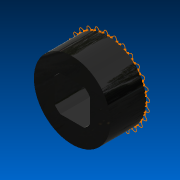
# Autodesk Inventor part: Versa Encoder Adapter
Saved by Autodesk Inventor 2022 (Build 260153000, 153)
## iProperties
Created: 2022-04-19
Part Number: Versa Encoder Adapter
Material: PET Plastic
Document SubType Name: Modeling
Designer: score_nygvs6w
Density: 1.541 g/cm^3
Appearance: Smooth - Black
Author: score_nygvs6w
Autodesk Inventor part; units mm, degrees
ref_plane "YZ Plane" through (0, 0, 0) normal (1, 0, 0) x (0, 1, 0)
ref_plane "XZ Plane" through (0, 0, 0) normal (0, 1, 0) x (-1, 0, 0)
ref_plane "XY Plane" through (0, 0, 0) normal (0, 0, 1) x (1, 0, 0)
sketch "Sketch1" plane through (0, 0, 0) normal (0, 0, 1) x (1, 0, 0)
  point P0 (0, 0)
sketch "Sketch2" plane through (0, 0, 0) normal (0, 0, 1) x (1, 0, 0)
  line L0 (-2.1061, 3.175) -> (2.1061, 3.175)
  line L1 (3.175, 2.1061) -> (3.175, -2.1061)
  line L2 (2.1061, -3.175) -> (-2.1061, -3.175)
  line L3 (-3.175, -2.1061) -> (-3.175, 2.1061)
  arc A0 (-2.1061, 3.175) -> (-3.175, 2.1061) centre (0, 0) ccw
  arc A1 (3.175, 2.1061) -> (2.1061, 3.175) centre (0, 0) ccw
  arc A2 (-3.175, -2.1061) -> (-2.1061, -3.175) centre (0, 0) ccw
  arc A3 (2.1061, -3.175) -> (3.175, -2.1061) centre (0, 0) ccw
  circle A4 centre (0, 0) radius 6.797
  dimension "d0" = 6.35
  dimension "d2" = 3.81
  dimension "d3" = 13.594
  constraints: 8 end point, 8 point on circle, 5 centre point, 4 perpendicular, 3 concentric, 2 coincident, 2 parallel, 1 horizontal
  measures "d0" distance between parallel lines of L1 L3
  measures "d2" radius of A2
  measures "d3" diameter of A4
extrude "Extrusion1" add sketch "Sketch2" along normal blind 6.35
sketch "Sketch3" plane through (0, 0, 0) normal (0, 0, -1) x (-1, 0, 0)
  arc A0 (5.3745, -4.161) -> (5.6838, -3.7274) centre (0, 0) ccw projected
  spline S0 degree 3 poles (5.6838, -3.7274) (5.7254, -3.7321) (5.7892, -3.7379) (5.876, -3.7432) (5.9447, -3.7461) (6.0157, -3.7477) (6.0892, -3.7479) (6.165, -3.7467) (6.2568, -3.7428) (6.3283, -3.7405) (6.3775, -3.7345) (6.39, -3.7308) (6.4012, -3.726) (6.4118, -3.7198) (6.4215, -3.7124) (6.4326, -3.7017) (6.4476, -3.6797) (6.4651, -3.6465) (6.4877, -3.6071) (6.5092, -3.5672) (6.5282, -3.5348) (6.539, -3.5104) (6.5422, -3.4953) (6.5434, -3.4831) (6.543, -3.4709) (6.5411, -3.4589) (6.5377, -3.4463) (6.5169, -3.4013) (6.4811, -3.3394) (6.436, -3.2593) (6.397, -3.1943) (6.3581, -3.132) (6.3192, -3.0725) (6.2805, -3.0157) (6.2301, -2.9448) (6.1916, -2.8937) (6.1656, -2.8608) knots 0.000063 0.000063 0.000063 0.000063 0.072335 0.110531 0.150078 0.190978 0.23323 0.276835 0.321791 0.391759 0.40017 0.407178 0.414186 0.421194 0.428201 0.435209 0.447802 0.473901 0.5 0.526099 0.552198 0.564791 0.571799 0.578806 0.585814 0.592822 0.59983 0.608241 0.678209 0.723165 0.76677 0.809022 0.849922 0.889469 0.927665 0.999937 0.999937 0.999937 0.999937 projected
  arc A1 (6.1656, -2.8608) -> (6.3707, -2.3692) centre (0, 0) ccw projected
  spline S1 degree 3 poles (6.3707, -2.3692) (6.4123, -2.3645) (6.4758, -2.3559) (6.5616, -2.3419) (6.6292, -2.3294) (6.6989, -2.3151) (6.7705, -2.299) (6.8442, -2.281) (6.9328, -2.2567) (7.0019, -2.2386) (7.0486, -2.2217) (7.0599, -2.2153) (7.0698, -2.2081) (7.0787, -2.1998) (7.0866, -2.1904) (7.0951, -2.1775) (7.1048, -2.1527) (7.1145, -2.1164) (7.1277, -2.073) (7.1398, -2.0293) (7.1511, -1.9935) (7.1562, -1.9673) (7.156, -1.9519) (7.1544, -1.9398) (7.1513, -1.9279) (7.1468, -1.9166) (7.1407, -1.9051) (7.1103, -1.8659) (7.0617, -1.8134) (6.9999, -1.7455) (6.9474, -1.6908) (6.8956, -1.6387) (6.8445, -1.5893) (6.7941, -1.5425) (6.7292, -1.4846) (6.6802, -1.4434) (6.6476, -1.4171) knots 0.000063 0.000063 0.000063 0.000063 0.072335 0.110531 0.150078 0.190978 0.23323 0.276835 0.321791 0.391759 0.40017 0.407178 0.414186 0.421194 0.428201 0.435209 0.447802 0.473901 0.5 0.526099 0.552198 0.564791 0.571799 0.578806 0.585814 0.592822 0.59983 0.608241 0.678209 0.723165 0.76677 0.809022 0.849922 0.889469 0.927665 0.999937 0.999937 0.999937 0.999937 projected
  arc A2 (6.6476, -1.4171) -> (6.7382, -0.8922) centre (0, 0) ccw projected
  spline S2 degree 3 poles (6.7382, -0.8922) (6.7777, -0.8783) (6.8377, -0.8559) (6.9182, -0.8231) (6.9813, -0.7959) (7.0461, -0.7665) (7.1123, -0.7347) (7.1801, -0.7008) (7.2611, -0.6575) (7.3245, -0.6244) (7.3662, -0.5976) (7.3759, -0.5888) (7.3839, -0.5796) (7.3908, -0.5695) (7.3963, -0.5586) (7.4017, -0.5441) (7.4056, -0.5178) (7.407, -0.4803) (7.4103, -0.435) (7.4123, -0.3897) (7.4154, -0.3523) (7.4145, -0.3256) (7.4109, -0.3106) (7.4066, -0.2991) (7.401, -0.2883) (7.3941, -0.2782) (7.3856, -0.2684) (7.3472, -0.2369) (7.2882, -0.1966) (7.2128, -0.1441) (7.1495, -0.1024) (7.0874, -0.0632) (7.0265, -0.0264) (6.967, 0.008) (6.8909, 0.05) (6.8339, 0.0793) (6.7963, 0.0977) knots 0.000063 0.000063 0.000063 0.000063 0.072335 0.110531 0.150078 0.190978 0.23323 0.276835 0.321791 0.391759 0.40017 0.407178 0.414186 0.421194 0.428201 0.435209 0.447802 0.473901 0.5 0.526099 0.552198 0.564791 0.571799 0.578806 0.585814 0.592822 0.59983 0.608241 0.678209 0.723165 0.76677 0.809022 0.849922 0.889469 0.927665 0.999937 0.999937 0.999937 0.999937 projected
  arc A3 (6.7963, 0.0977) -> (6.7678, 0.6296) centre (0, 0) ccw projected
  spline S3 degree 3 poles (6.7678, 0.6296) (6.8032, 0.6519) (6.8567, 0.6871) (6.9279, 0.737) (6.9834, 0.7776) (7.04, 0.8207) (7.0975, 0.8663) (7.1561, 0.9145) (7.2254, 0.9748) (7.2798, 1.0212) (7.3145, 1.0566) (7.322, 1.0673) (7.3278, 1.078) (7.3322, 1.0894) (7.3352, 1.1012) (7.3372, 1.1166) (7.3352, 1.1431) (7.3282, 1.18) (7.3213, 1.2249) (7.3132, 1.2695) (7.3078, 1.3067) (7.3011, 1.3324) (7.2942, 1.3463) (7.2875, 1.3565) (7.2796, 1.3658) (7.2706, 1.3741) (7.2601, 1.3818) (7.2157, 1.404) (7.1492, 1.4301) (7.064, 1.4645) (6.993, 1.491) (6.9237, 1.5155) (6.8562, 1.5378) (6.7905, 1.5581) (6.707, 1.5821) (6.6449, 1.598) (6.6042, 1.6076) knots 0.000063 0.000063 0.000063 0.000063 0.072335 0.110531 0.150078 0.190978 0.23323 0.276835 0.321791 0.391759 0.40017 0.407178 0.414186 0.421194 0.428201 0.435209 0.447802 0.473901 0.5 0.526099 0.552198 0.564791 0.571799 0.578806 0.585814 0.592822 0.59983 0.608241 0.678209 0.723165 0.76677 0.809022 0.849922 0.889469 0.927665 0.999937 0.999937 0.999937 0.999937 projected
  arc A4 (6.6042, 1.6076) -> (6.458, 2.1198) centre (0, 0) ccw projected
  spline S4 degree 3 poles (6.458, 2.1198) (6.4876, 2.1494) (6.5319, 2.1956) (6.5902, 2.2601) (6.6353, 2.312) (6.6809, 2.3666) (6.7268, 2.4239) (6.7731, 2.4839) (6.8273, 2.5581) (6.87, 2.6155) (6.896, 2.6577) (6.9009, 2.6698) (6.9042, 2.6816) (6.9059, 2.6936) (6.9062, 2.7058) (6.9048, 2.7213) (6.8969, 2.7467) (6.8819, 2.7811) (6.8652, 2.8233) (6.8474, 2.865) (6.8338, 2.9) (6.8216, 2.9237) (6.8117, 2.9356) (6.8029, 2.9441) (6.7932, 2.9514) (6.7826, 2.9575) (6.7706, 2.9627) (6.7224, 2.9744) (6.6517, 2.9851) (6.561, 2.9997) (6.4859, 3.0097) (6.4129, 3.0182) (6.3421, 3.0249) (6.2736, 3.0301) (6.1867, 3.0349) (6.1227, 3.0366) (6.0809, 3.0368) knots 0.000063 0.000063 0.000063 0.000063 0.072335 0.110531 0.150078 0.190978 0.23323 0.276835 0.321791 0.391759 0.40017 0.407178 0.414186 0.421194 0.428201 0.435209 0.447802 0.473901 0.5 0.526099 0.552198 0.564791 0.571799 0.578806 0.585814 0.592822 0.59983 0.608241 0.678209 0.723165 0.76677 0.809022 0.849922 0.889469 0.927665 0.999937 0.999937 0.999937 0.999937 projected
  arc A5 (6.0809, 3.0368) -> (5.8244, 3.5036) centre (0, 0) ccw projected
  spline S5 degree 3 poles (5.8244, 3.5036) (5.8466, 3.5391) (5.8795, 3.5941) (5.922, 3.6699) (5.9544, 3.7306) (5.9867, 3.7939) (6.0188, 3.86) (6.0506, 3.9288) (6.0869, 4.0132) (6.1158, 4.0786) (6.1317, 4.1256) (6.1338, 4.1385) (6.1344, 4.1506) (6.1334, 4.1628) (6.131, 4.1748) (6.1261, 4.1895) (6.1128, 4.2125) (6.0905, 4.2427) (6.0648, 4.2802) (6.0382, 4.3169) (6.0172, 4.348) (5.9999, 4.3683) (5.9877, 4.3778) (5.9772, 4.3841) (5.9661, 4.3891) (5.9544, 4.3926) (5.9416, 4.395) (5.892, 4.3957) (5.8207, 4.3904) (5.729, 4.3845) (5.6535, 4.3775) (5.5805, 4.3695) (5.51, 4.3603) (5.442, 4.3501) (5.3563, 4.3355) (5.2935, 4.3229) (5.2526, 4.3138) knots 0.000063 0.000063 0.000063 0.000063 0.072335 0.110531 0.150078 0.190978 0.23323 0.276835 0.321791 0.391759 0.40017 0.407178 0.414186 0.421194 0.428201 0.435209 0.447802 0.473901 0.5 0.526099 0.552198 0.564791 0.571799 0.578806 0.585814 0.592822 0.59983 0.608241 0.678209 0.723165 0.76677 0.809022 0.849922 0.889469 0.927665 0.999937 0.999937 0.999937 0.999937 projected
  arc A6 (5.2526, 4.3138) -> (4.8987, 4.7119) centre (0, 0) ccw projected
  spline S6 degree 3 poles (4.8987, 4.7119) (4.9125, 4.7514) (4.9324, 4.8123) (4.9569, 4.8957) (4.975, 4.962) (4.9924, 5.031) (5.0089, 5.1025) (5.0246, 5.1767) (5.0413, 5.2671) (5.0549, 5.3372) (5.06, 5.3866) (5.0591, 5.3996) (5.0569, 5.4116) (5.0533, 5.4233) (5.0483, 5.4344) (5.0403, 5.4476) (5.0221, 5.4672) (4.9937, 5.4916) (4.9603, 5.5224) (4.9262, 5.5523) (4.8988, 5.5779) (4.8775, 5.5939) (4.8634, 5.6004) (4.8518, 5.6042) (4.8399, 5.6066) (4.8277, 5.6075) (4.8146, 5.6069) (4.7661, 5.5966) (4.6978, 5.5756) (4.6098, 5.5494) (4.5377, 5.5258) (4.4683, 5.5017) (4.4016, 5.4771) (4.3376, 5.452) (4.2573, 5.4187) (4.1989, 5.3924) (4.161, 5.3745) knots 0.000063 0.000063 0.000063 0.000063 0.072335 0.110531 0.150078 0.190978 0.23323 0.276835 0.321791 0.391759 0.40017 0.407178 0.414186 0.421194 0.428201 0.435209 0.447802 0.473901 0.5 0.526099 0.552198 0.564791 0.571799 0.578806 0.585814 0.592822 0.59983 0.608241 0.678209 0.723165 0.76677 0.809022 0.849922 0.889469 0.927665 0.999937 0.999937 0.999937 0.999937 projected
  arc A7 (4.161, 5.3745) -> (3.7274, 5.6838) centre (0, 0) ccw projected
  spline S7 degree 3 poles (3.7274, 5.6838) (3.7321, 5.7254) (3.7379, 5.7892) (3.7432, 5.876) (3.7461, 5.9447) (3.7477, 6.0157) (3.7479, 6.0892) (3.7467, 6.165) (3.7428, 6.2568) (3.7405, 6.3283) (3.7345, 6.3775) (3.7308, 6.39) (3.726, 6.4012) (3.7198, 6.4118) (3.7124, 6.4215) (3.7017, 6.4326) (3.6797, 6.4476) (3.6465, 6.4651) (3.6071, 6.4877) (3.5672, 6.5092) (3.5348, 6.5282) (3.5104, 6.539) (3.4953, 6.5422) (3.4831, 6.5434) (3.4709, 6.543) (3.4589, 6.5411) (3.4463, 6.5377) (3.4013, 6.5169) (3.3394, 6.4811) (3.2593, 6.436) (3.1943, 6.397) (3.132, 6.3581) (3.0725, 6.3192) (3.0157, 6.2805) (2.9448, 6.2301) (2.8937, 6.1916) (2.8608, 6.1656) knots 0.000063 0.000063 0.000063 0.000063 0.072335 0.110531 0.150078 0.190978 0.23323 0.276835 0.321791 0.391759 0.40017 0.407178 0.414186 0.421194 0.428201 0.435209 0.447802 0.473901 0.5 0.526099 0.552198 0.564791 0.571799 0.578806 0.585814 0.592822 0.59983 0.608241 0.678209 0.723165 0.76677 0.809022 0.849922 0.889469 0.927665 0.999937 0.999937 0.999937 0.999937 projected
  arc A8 (2.8608, 6.1656) -> (2.3692, 6.3707) centre (0, 0) ccw projected
  spline S8 degree 3 poles (2.3692, 6.3707) (2.3645, 6.4123) (2.3559, 6.4758) (2.3419, 6.5616) (2.3294, 6.6292) (2.3151, 6.6989) (2.299, 6.7705) (2.281, 6.8442) (2.2567, 6.9328) (2.2386, 7.0019) (2.2217, 7.0486) (2.2153, 7.0599) (2.2081, 7.0698) (2.1998, 7.0787) (2.1904, 7.0866) (2.1775, 7.0951) (2.1527, 7.1048) (2.1164, 7.1145) (2.073, 7.1277) (2.0293, 7.1398) (1.9935, 7.1511) (1.9673, 7.1562) (1.9519, 7.156) (1.9398, 7.1544) (1.9279, 7.1513) (1.9166, 7.1468) (1.9051, 7.1407) (1.8659, 7.1103) (1.8134, 7.0617) (1.7455, 6.9999) (1.6908, 6.9474) (1.6387, 6.8956) (1.5893, 6.8445) (1.5425, 6.7941) (1.4846, 6.7292) (1.4434, 6.6802) (1.4171, 6.6476) knots 0.000063 0.000063 0.000063 0.000063 0.072335 0.110531 0.150078 0.190978 0.23323 0.276835 0.321791 0.391759 0.40017 0.407178 0.414186 0.421194 0.428201 0.435209 0.447802 0.473901 0.5 0.526099 0.552198 0.564791 0.571799 0.578806 0.585814 0.592822 0.59983 0.608241 0.678209 0.723165 0.76677 0.809022 0.849922 0.889469 0.927665 0.999937 0.999937 0.999937 0.999937 projected
  arc A9 (1.4171, 6.6476) -> (0.8922, 6.7382) centre (0, 0) ccw projected
  spline S9 degree 3 poles (0.8922, 6.7382) (0.8783, 6.7777) (0.8559, 6.8377) (0.8231, 6.9182) (0.7959, 6.9813) (0.7665, 7.0461) (0.7347, 7.1123) (0.7008, 7.1801) (0.6575, 7.2611) (0.6244, 7.3245) (0.5976, 7.3662) (0.5888, 7.3759) (0.5796, 7.3839) (0.5695, 7.3908) (0.5586, 7.3963) (0.5441, 7.4017) (0.5178, 7.4056) (0.4803, 7.407) (0.435, 7.4103) (0.3897, 7.4123) (0.3523, 7.4154) (0.3256, 7.4145) (0.3106, 7.4109) (0.2991, 7.4066) (0.2883, 7.401) (0.2782, 7.3941) (0.2684, 7.3856) (0.2369, 7.3472) (0.1966, 7.2882) (0.1441, 7.2128) (0.1024, 7.1495) (0.0632, 7.0874) (0.0264, 7.0265) (-0.008, 6.967) (-0.05, 6.8909) (-0.0793, 6.8339) (-0.0977, 6.7963) knots 0.000063 0.000063 0.000063 0.000063 0.072335 0.110531 0.150078 0.190978 0.23323 0.276835 0.321791 0.391759 0.40017 0.407178 0.414186 0.421194 0.428201 0.435209 0.447802 0.473901 0.5 0.526099 0.552198 0.564791 0.571799 0.578806 0.585814 0.592822 0.59983 0.608241 0.678209 0.723165 0.76677 0.809022 0.849922 0.889469 0.927665 0.999937 0.999937 0.999937 0.999937 projected
  arc A10 (-0.0977, 6.7963) -> (-0.6296, 6.7678) centre (0, 0) ccw projected
  spline S10 degree 3 poles (-0.6296, 6.7678) (-0.6519, 6.8032) (-0.6871, 6.8567) (-0.737, 6.9279) (-0.7776, 6.9834) (-0.8207, 7.04) (-0.8663, 7.0975) (-0.9145, 7.1561) (-0.9748, 7.2254) (-1.0212, 7.2798) (-1.0566, 7.3145) (-1.0673, 7.322) (-1.078, 7.3278) (-1.0894, 7.3322) (-1.1012, 7.3352) (-1.1166, 7.3372) (-1.1431, 7.3352) (-1.18, 7.3282) (-1.2249, 7.3213) (-1.2695, 7.3132) (-1.3067, 7.3078) (-1.3324, 7.3011) (-1.3463, 7.2942) (-1.3565, 7.2875) (-1.3658, 7.2796) (-1.3741, 7.2706) (-1.3818, 7.2601) (-1.404, 7.2157) (-1.4301, 7.1492) (-1.4645, 7.064) (-1.491, 6.993) (-1.5155, 6.9237) (-1.5378, 6.8562) (-1.5581, 6.7905) (-1.5821, 6.707) (-1.598, 6.6449) (-1.6076, 6.6042) knots 0.000063 0.000063 0.000063 0.000063 0.072335 0.110531 0.150078 0.190978 0.23323 0.276835 0.321791 0.391759 0.40017 0.407178 0.414186 0.421194 0.428201 0.435209 0.447802 0.473901 0.5 0.526099 0.552198 0.564791 0.571799 0.578806 0.585814 0.592822 0.59983 0.608241 0.678209 0.723165 0.76677 0.809022 0.849922 0.889469 0.927665 0.999937 0.999937 0.999937 0.999937 projected
  arc A11 (-1.6076, 6.6042) -> (-2.1198, 6.458) centre (0, 0) ccw projected
  spline S11 degree 3 poles (-2.1198, 6.458) (-2.1494, 6.4876) (-2.1956, 6.5319) (-2.2601, 6.5902) (-2.312, 6.6353) (-2.3666, 6.6809) (-2.4239, 6.7268) (-2.4839, 6.7731) (-2.5581, 6.8273) (-2.6155, 6.87) (-2.6577, 6.896) (-2.6698, 6.9009) (-2.6816, 6.9042) (-2.6936, 6.9059) (-2.7058, 6.9062) (-2.7213, 6.9048) (-2.7467, 6.8969) (-2.7811, 6.8819) (-2.8233, 6.8652) (-2.865, 6.8474) (-2.9, 6.8338) (-2.9237, 6.8216) (-2.9356, 6.8117) (-2.9441, 6.8029) (-2.9514, 6.7932) (-2.9575, 6.7826) (-2.9627, 6.7706) (-2.9744, 6.7224) (-2.9851, 6.6517) (-2.9997, 6.561) (-3.0097, 6.4859) (-3.0182, 6.4129) (-3.0249, 6.3421) (-3.0301, 6.2736) (-3.0349, 6.1867) (-3.0366, 6.1227) (-3.0368, 6.0809) knots 0.000063 0.000063 0.000063 0.000063 0.072335 0.110531 0.150078 0.190978 0.23323 0.276835 0.321791 0.391759 0.40017 0.407178 0.414186 0.421194 0.428201 0.435209 0.447802 0.473901 0.5 0.526099 0.552198 0.564791 0.571799 0.578806 0.585814 0.592822 0.59983 0.608241 0.678209 0.723165 0.76677 0.809022 0.849922 0.889469 0.927665 0.999937 0.999937 0.999937 0.999937 projected
  arc A12 (-3.0368, 6.0809) -> (-3.5036, 5.8244) centre (0, 0) ccw projected
  spline S12 degree 3 poles (-3.5036, 5.8244) (-3.5391, 5.8466) (-3.5941, 5.8795) (-3.6699, 5.922) (-3.7306, 5.9544) (-3.7939, 5.9867) (-3.86, 6.0188) (-3.9288, 6.0506) (-4.0132, 6.0869) (-4.0786, 6.1158) (-4.1256, 6.1317) (-4.1385, 6.1338) (-4.1506, 6.1344) (-4.1628, 6.1334) (-4.1748, 6.131) (-4.1895, 6.1261) (-4.2125, 6.1128) (-4.2427, 6.0905) (-4.2802, 6.0648) (-4.3169, 6.0382) (-4.348, 6.0172) (-4.3683, 5.9999) (-4.3778, 5.9877) (-4.3841, 5.9772) (-4.3891, 5.9661) (-4.3926, 5.9544) (-4.395, 5.9416) (-4.3957, 5.892) (-4.3904, 5.8207) (-4.3845, 5.729) (-4.3775, 5.6535) (-4.3695, 5.5805) (-4.3603, 5.51) (-4.3501, 5.442) (-4.3355, 5.3563) (-4.3229, 5.2935) (-4.3138, 5.2526) knots 0.000063 0.000063 0.000063 0.000063 0.072335 0.110531 0.150078 0.190978 0.23323 0.276835 0.321791 0.391759 0.40017 0.407178 0.414186 0.421194 0.428201 0.435209 0.447802 0.473901 0.5 0.526099 0.552198 0.564791 0.571799 0.578806 0.585814 0.592822 0.59983 0.608241 0.678209 0.723165 0.76677 0.809022 0.849922 0.889469 0.927665 0.999937 0.999937 0.999937 0.999937 projected
  arc A13 (-4.3138, 5.2526) -> (-4.7119, 4.8987) centre (0, 0) ccw projected
  spline S13 degree 3 poles (-4.7119, 4.8987) (-4.7514, 4.9125) (-4.8123, 4.9324) (-4.8957, 4.9569) (-4.962, 4.975) (-5.031, 4.9924) (-5.1025, 5.0089) (-5.1767, 5.0246) (-5.2671, 5.0413) (-5.3372, 5.0549) (-5.3866, 5.06) (-5.3996, 5.0591) (-5.4116, 5.0569) (-5.4233, 5.0533) (-5.4344, 5.0483) (-5.4476, 5.0403) (-5.4672, 5.0221) (-5.4916, 4.9937) (-5.5224, 4.9603) (-5.5523, 4.9262) (-5.5779, 4.8988) (-5.5939, 4.8775) (-5.6004, 4.8634) (-5.6042, 4.8518) (-5.6066, 4.8399) (-5.6075, 4.8277) (-5.6069, 4.8146) (-5.5966, 4.7661) (-5.5756, 4.6978) (-5.5494, 4.6098) (-5.5258, 4.5377) (-5.5017, 4.4683) (-5.4771, 4.4016) (-5.452, 4.3376) (-5.4187, 4.2573) (-5.3924, 4.1989) (-5.3745, 4.161) knots 0.000063 0.000063 0.000063 0.000063 0.072335 0.110531 0.150078 0.190978 0.23323 0.276835 0.321791 0.391759 0.40017 0.407178 0.414186 0.421194 0.428201 0.435209 0.447802 0.473901 0.5 0.526099 0.552198 0.564791 0.571799 0.578806 0.585814 0.592822 0.59983 0.608241 0.678209 0.723165 0.76677 0.809022 0.849922 0.889469 0.927665 0.999937 0.999937 0.999937 0.999937 projected
  arc A14 (-5.3745, 4.161) -> (-5.6838, 3.7274) centre (0, 0) ccw projected
  spline S14 degree 3 poles (-5.6838, 3.7274) (-5.7254, 3.7321) (-5.7892, 3.7379) (-5.876, 3.7432) (-5.9447, 3.7461) (-6.0157, 3.7477) (-6.0892, 3.7479) (-6.165, 3.7467) (-6.2568, 3.7428) (-6.3283, 3.7405) (-6.3775, 3.7345) (-6.39, 3.7308) (-6.4012, 3.726) (-6.4118, 3.7198) (-6.4215, 3.7124) (-6.4326, 3.7017) (-6.4476, 3.6797) (-6.4651, 3.6465) (-6.4877, 3.6071) (-6.5092, 3.5672) (-6.5282, 3.5348) (-6.539, 3.5104) (-6.5422, 3.4953) (-6.5434, 3.4831) (-6.543, 3.4709) (-6.5411, 3.4589) (-6.5377, 3.4463) (-6.5169, 3.4013) (-6.4811, 3.3394) (-6.436, 3.2593) (-6.397, 3.1943) (-6.3581, 3.132) (-6.3192, 3.0725) (-6.2805, 3.0157) (-6.2301, 2.9448) (-6.1916, 2.8937) (-6.1656, 2.8608) knots 0.000063 0.000063 0.000063 0.000063 0.072335 0.110531 0.150078 0.190978 0.23323 0.276835 0.321791 0.391759 0.40017 0.407178 0.414186 0.421194 0.428201 0.435209 0.447802 0.473901 0.5 0.526099 0.552198 0.564791 0.571799 0.578806 0.585814 0.592822 0.59983 0.608241 0.678209 0.723165 0.76677 0.809022 0.849922 0.889469 0.927665 0.999937 0.999937 0.999937 0.999937 projected
  arc A15 (-6.1656, 2.8608) -> (-6.3707, 2.3692) centre (0, 0) ccw projected
  spline S15 degree 3 poles (-6.3707, 2.3692) (-6.4123, 2.3645) (-6.4758, 2.3559) (-6.5616, 2.3419) (-6.6292, 2.3294) (-6.6989, 2.3151) (-6.7705, 2.299) (-6.8442, 2.281) (-6.9328, 2.2567) (-7.0019, 2.2386) (-7.0486, 2.2217) (-7.0599, 2.2153) (-7.0698, 2.2081) (-7.0787, 2.1998) (-7.0866, 2.1904) (-7.0951, 2.1775) (-7.1048, 2.1527) (-7.1145, 2.1164) (-7.1277, 2.073) (-7.1398, 2.0293) (-7.1511, 1.9935) (-7.1562, 1.9673) (-7.156, 1.9519) (-7.1544, 1.9398) (-7.1513, 1.9279) (-7.1468, 1.9166) (-7.1407, 1.9051) (-7.1103, 1.8659) (-7.0617, 1.8134) (-6.9999, 1.7455) (-6.9474, 1.6908) (-6.8956, 1.6387) (-6.8445, 1.5893) (-6.7941, 1.5425) (-6.7292, 1.4846) (-6.6802, 1.4434) (-6.6476, 1.4171) knots 0.000063 0.000063 0.000063 0.000063 0.072335 0.110531 0.150078 0.190978 0.23323 0.276835 0.321791 0.391759 0.40017 0.407178 0.414186 0.421194 0.428201 0.435209 0.447802 0.473901 0.5 0.526099 0.552198 0.564791 0.571799 0.578806 0.585814 0.592822 0.59983 0.608241 0.678209 0.723165 0.76677 0.809022 0.849922 0.889469 0.927665 0.999937 0.999937 0.999937 0.999937 projected
  arc A16 (-6.6476, 1.4171) -> (-6.7382, 0.8922) centre (0, 0) ccw projected
  spline S16 degree 3 poles (-6.7382, 0.8922) (-6.7777, 0.8783) (-6.8377, 0.8559) (-6.9182, 0.8231) (-6.9813, 0.7959) (-7.0461, 0.7665) (-7.1123, 0.7347) (-7.1801, 0.7008) (-7.2611, 0.6575) (-7.3245, 0.6244) (-7.3662, 0.5976) (-7.3759, 0.5888) (-7.3839, 0.5796) (-7.3908, 0.5695) (-7.3963, 0.5586) (-7.4017, 0.5441) (-7.4056, 0.5178) (-7.407, 0.4803) (-7.4103, 0.435) (-7.4123, 0.3897) (-7.4154, 0.3523) (-7.4145, 0.3256) (-7.4109, 0.3106) (-7.4066, 0.2991) (-7.401, 0.2883) (-7.3941, 0.2782) (-7.3856, 0.2684) (-7.3472, 0.2369) (-7.2882, 0.1966) (-7.2128, 0.1441) (-7.1495, 0.1024) (-7.0874, 0.0632) (-7.0265, 0.0264) (-6.967, -0.008) (-6.8909, -0.05) (-6.8339, -0.0793) (-6.7963, -0.0977) knots 0.000063 0.000063 0.000063 0.000063 0.072335 0.110531 0.150078 0.190978 0.23323 0.276835 0.321791 0.391759 0.40017 0.407178 0.414186 0.421194 0.428201 0.435209 0.447802 0.473901 0.5 0.526099 0.552198 0.564791 0.571799 0.578806 0.585814 0.592822 0.59983 0.608241 0.678209 0.723165 0.76677 0.809022 0.849922 0.889469 0.927665 0.999937 0.999937 0.999937 0.999937 projected
  arc A17 (-6.7963, -0.0977) -> (-6.7678, -0.6296) centre (0, 0) ccw projected
  spline S17 degree 3 poles (-6.7678, -0.6296) (-6.8032, -0.6519) (-6.8567, -0.6871) (-6.9279, -0.737) (-6.9834, -0.7776) (-7.04, -0.8207) (-7.0975, -0.8663) (-7.1561, -0.9145) (-7.2254, -0.9748) (-7.2798, -1.0212) (-7.3145, -1.0566) (-7.322, -1.0673) (-7.3278, -1.078) (-7.3322, -1.0894) (-7.3352, -1.1012) (-7.3372, -1.1166) (-7.3352, -1.1431) (-7.3282, -1.18) (-7.3213, -1.2249) (-7.3132, -1.2695) (-7.3078, -1.3067) (-7.3011, -1.3324) (-7.2942, -1.3463) (-7.2875, -1.3565) (-7.2796, -1.3658) (-7.2706, -1.3741) (-7.2601, -1.3818) (-7.2157, -1.404) (-7.1492, -1.4301) (-7.064, -1.4645) (-6.993, -1.491) (-6.9237, -1.5155) (-6.8562, -1.5378) (-6.7905, -1.5581) (-6.707, -1.5821) (-6.6449, -1.598) (-6.6042, -1.6076) knots 0.000063 0.000063 0.000063 0.000063 0.072335 0.110531 0.150078 0.190978 0.23323 0.276835 0.321791 0.391759 0.40017 0.407178 0.414186 0.421194 0.428201 0.435209 0.447802 0.473901 0.5 0.526099 0.552198 0.564791 0.571799 0.578806 0.585814 0.592822 0.59983 0.608241 0.678209 0.723165 0.76677 0.809022 0.849922 0.889469 0.927665 0.999937 0.999937 0.999937 0.999937 projected
  arc A18 (-6.6042, -1.6076) -> (-6.458, -2.1198) centre (0, 0) ccw projected
  spline S18 degree 3 poles (-6.458, -2.1198) (-6.4876, -2.1494) (-6.5319, -2.1956) (-6.5902, -2.2601) (-6.6353, -2.312) (-6.6809, -2.3666) (-6.7268, -2.4239) (-6.7731, -2.4839) (-6.8273, -2.5581) (-6.87, -2.6155) (-6.896, -2.6577) (-6.9009, -2.6698) (-6.9042, -2.6816) (-6.9059, -2.6936) (-6.9062, -2.7058) (-6.9048, -2.7213) (-6.8969, -2.7467) (-6.8819, -2.7811) (-6.8652, -2.8233) (-6.8474, -2.865) (-6.8338, -2.9) (-6.8216, -2.9237) (-6.8117, -2.9356) (-6.8029, -2.9441) (-6.7932, -2.9514) (-6.7826, -2.9575) (-6.7706, -2.9627) (-6.7224, -2.9744) (-6.6517, -2.9851) (-6.561, -2.9997) (-6.4859, -3.0097) (-6.4129, -3.0182) (-6.3421, -3.0249) (-6.2736, -3.0301) (-6.1867, -3.0349) (-6.1227, -3.0366) (-6.0809, -3.0368) knots 0.000063 0.000063 0.000063 0.000063 0.072335 0.110531 0.150078 0.190978 0.23323 0.276835 0.321791 0.391759 0.40017 0.407178 0.414186 0.421194 0.428201 0.435209 0.447802 0.473901 0.5 0.526099 0.552198 0.564791 0.571799 0.578806 0.585814 0.592822 0.59983 0.608241 0.678209 0.723165 0.76677 0.809022 0.849922 0.889469 0.927665 0.999937 0.999937 0.999937 0.999937 projected
  arc A19 (-6.0809, -3.0368) -> (-5.8244, -3.5036) centre (0, 0) ccw projected
  spline S19 degree 3 poles (-5.8244, -3.5036) (-5.8466, -3.5391) (-5.8795, -3.5941) (-5.922, -3.6699) (-5.9544, -3.7306) (-5.9867, -3.7939) (-6.0188, -3.86) (-6.0506, -3.9288) (-6.0869, -4.0132) (-6.1158, -4.0786) (-6.1317, -4.1256) (-6.1338, -4.1385) (-6.1344, -4.1506) (-6.1334, -4.1628) (-6.131, -4.1748) (-6.1261, -4.1895) (-6.1128, -4.2125) (-6.0905, -4.2427) (-6.0648, -4.2802) (-6.0382, -4.3169) (-6.0172, -4.348) (-5.9999, -4.3683) (-5.9877, -4.3778) (-5.9772, -4.3841) (-5.9661, -4.3891) (-5.9544, -4.3926) (-5.9416, -4.395) (-5.892, -4.3957) (-5.8207, -4.3904) (-5.729, -4.3845) (-5.6535, -4.3775) (-5.5805, -4.3695) (-5.51, -4.3603) (-5.442, -4.3501) (-5.3563, -4.3355) (-5.2935, -4.3229) (-5.2526, -4.3138) knots 0.000063 0.000063 0.000063 0.000063 0.072335 0.110531 0.150078 0.190978 0.23323 0.276835 0.321791 0.391759 0.40017 0.407178 0.414186 0.421194 0.428201 0.435209 0.447802 0.473901 0.5 0.526099 0.552198 0.564791 0.571799 0.578806 0.585814 0.592822 0.59983 0.608241 0.678209 0.723165 0.76677 0.809022 0.849922 0.889469 0.927665 0.999937 0.999937 0.999937 0.999937 projected
  arc A20 (-5.2526, -4.3138) -> (-4.8987, -4.7119) centre (0, 0) ccw projected
  spline S20 degree 3 poles (-4.8987, -4.7119) (-4.9125, -4.7514) (-4.9324, -4.8123) (-4.9569, -4.8957) (-4.975, -4.962) (-4.9924, -5.031) (-5.0089, -5.1025) (-5.0246, -5.1767) (-5.0413, -5.2671) (-5.0549, -5.3372) (-5.06, -5.3866) (-5.0591, -5.3996) (-5.0569, -5.4116) (-5.0533, -5.4233) (-5.0483, -5.4344) (-5.0403, -5.4476) (-5.0221, -5.4672) (-4.9937, -5.4916) (-4.9603, -5.5224) (-4.9262, -5.5523) (-4.8988, -5.5779) (-4.8775, -5.5939) (-4.8634, -5.6004) (-4.8518, -5.6042) (-4.8399, -5.6066) (-4.8277, -5.6075) (-4.8146, -5.6069) (-4.7661, -5.5966) (-4.6978, -5.5756) (-4.6098, -5.5494) (-4.5377, -5.5258) (-4.4683, -5.5017) (-4.4016, -5.4771) (-4.3376, -5.452) (-4.2573, -5.4187) (-4.1989, -5.3924) (-4.161, -5.3745) knots 0.000063 0.000063 0.000063 0.000063 0.072335 0.110531 0.150078 0.190978 0.23323 0.276835 0.321791 0.391759 0.40017 0.407178 0.414186 0.421194 0.428201 0.435209 0.447802 0.473901 0.5 0.526099 0.552198 0.564791 0.571799 0.578806 0.585814 0.592822 0.59983 0.608241 0.678209 0.723165 0.76677 0.809022 0.849922 0.889469 0.927665 0.999937 0.999937 0.999937 0.999937 projected
  arc A21 (-4.161, -5.3745) -> (-3.7274, -5.6838) centre (0, 0) ccw projected
  spline S21 degree 3 poles (-3.7274, -5.6838) (-3.7321, -5.7254) (-3.7379, -5.7892) (-3.7432, -5.876) (-3.7461, -5.9447) (-3.7477, -6.0157) (-3.7479, -6.0892) (-3.7467, -6.165) (-3.7428, -6.2568) (-3.7405, -6.3283) (-3.7345, -6.3775) (-3.7308, -6.39) (-3.726, -6.4012) (-3.7198, -6.4118) (-3.7124, -6.4215) (-3.7017, -6.4326) (-3.6797, -6.4476) (-3.6465, -6.4651) (-3.6071, -6.4877) (-3.5672, -6.5092) (-3.5348, -6.5282) (-3.5104, -6.539) (-3.4953, -6.5422) (-3.4831, -6.5434) (-3.4709, -6.543) (-3.4589, -6.5411) (-3.4463, -6.5377) (-3.4013, -6.5169) (-3.3394, -6.4811) (-3.2593, -6.436) (-3.1943, -6.397) (-3.132, -6.3581) (-3.0725, -6.3192) (-3.0157, -6.2805) (-2.9448, -6.2301) (-2.8937, -6.1916) (-2.8608, -6.1656) knots 0.000063 0.000063 0.000063 0.000063 0.072335 0.110531 0.150078 0.190978 0.23323 0.276835 0.321791 0.391759 0.40017 0.407178 0.414186 0.421194 0.428201 0.435209 0.447802 0.473901 0.5 0.526099 0.552198 0.564791 0.571799 0.578806 0.585814 0.592822 0.59983 0.608241 0.678209 0.723165 0.76677 0.809022 0.849922 0.889469 0.927665 0.999937 0.999937 0.999937 0.999937 projected
  arc A22 (-2.8608, -6.1656) -> (-2.3692, -6.3707) centre (0, 0) ccw projected
  spline S22 degree 3 poles (-2.3692, -6.3707) (-2.3645, -6.4123) (-2.3559, -6.4758) (-2.3419, -6.5616) (-2.3294, -6.6292) (-2.3151, -6.6989) (-2.299, -6.7705) (-2.281, -6.8442) (-2.2567, -6.9328) (-2.2386, -7.0019) (-2.2217, -7.0486) (-2.2153, -7.0599) (-2.2081, -7.0698) (-2.1998, -7.0787) (-2.1904, -7.0866) (-2.1775, -7.0951) (-2.1527, -7.1048) (-2.1164, -7.1145) (-2.073, -7.1277) (-2.0293, -7.1398) (-1.9935, -7.1511) (-1.9673, -7.1562) (-1.9519, -7.156) (-1.9398, -7.1544) (-1.9279, -7.1513) (-1.9166, -7.1468) (-1.9051, -7.1407) (-1.8659, -7.1103) (-1.8134, -7.0617) (-1.7455, -6.9999) (-1.6908, -6.9474) (-1.6387, -6.8956) (-1.5893, -6.8445) (-1.5425, -6.7941) (-1.4846, -6.7292) (-1.4434, -6.6802) (-1.4171, -6.6476) knots 0.000063 0.000063 0.000063 0.000063 0.072335 0.110531 0.150078 0.190978 0.23323 0.276835 0.321791 0.391759 0.40017 0.407178 0.414186 0.421194 0.428201 0.435209 0.447802 0.473901 0.5 0.526099 0.552198 0.564791 0.571799 0.578806 0.585814 0.592822 0.59983 0.608241 0.678209 0.723165 0.76677 0.809022 0.849922 0.889469 0.927665 0.999937 0.999937 0.999937 0.999937 projected
  arc A23 (-1.4171, -6.6476) -> (-0.8922, -6.7382) centre (0, 0) ccw projected
  spline S23 degree 3 poles (-0.8922, -6.7382) (-0.8783, -6.7777) (-0.8559, -6.8377) (-0.8231, -6.9182) (-0.7959, -6.9813) (-0.7665, -7.0461) (-0.7347, -7.1123) (-0.7008, -7.1801) (-0.6575, -7.2611) (-0.6244, -7.3245) (-0.5976, -7.3662) (-0.5888, -7.3759) (-0.5796, -7.3839) (-0.5695, -7.3908) (-0.5586, -7.3963) (-0.5441, -7.4017) (-0.5178, -7.4056) (-0.4803, -7.407) (-0.435, -7.4103) (-0.3897, -7.4123) (-0.3523, -7.4154) (-0.3256, -7.4145) (-0.3106, -7.4109) (-0.2991, -7.4066) (-0.2883, -7.401) (-0.2782, -7.3941) (-0.2684, -7.3856) (-0.2369, -7.3472) (-0.1966, -7.2882) (-0.1441, -7.2128) (-0.1024, -7.1495) (-0.0632, -7.0874) (-0.0264, -7.0265) (0.008, -6.967) (0.05, -6.8909) (0.0793, -6.8339) (0.0977, -6.7963) knots 0.000063 0.000063 0.000063 0.000063 0.072335 0.110531 0.150078 0.190978 0.23323 0.276835 0.321791 0.391759 0.40017 0.407178 0.414186 0.421194 0.428201 0.435209 0.447802 0.473901 0.5 0.526099 0.552198 0.564791 0.571799 0.578806 0.585814 0.592822 0.59983 0.608241 0.678209 0.723165 0.76677 0.809022 0.849922 0.889469 0.927665 0.999937 0.999937 0.999937 0.999937 projected
  arc A24 (0.0977, -6.7963) -> (0.6296, -6.7678) centre (0, 0) ccw projected
  spline S24 degree 3 poles (0.6296, -6.7678) (0.6519, -6.8032) (0.6871, -6.8567) (0.737, -6.9279) (0.7776, -6.9834) (0.8207, -7.04) (0.8663, -7.0975) (0.9145, -7.1561) (0.9748, -7.2254) (1.0212, -7.2798) (1.0566, -7.3145) (1.0673, -7.322) (1.078, -7.3278) (1.0894, -7.3322) (1.1012, -7.3352) (1.1166, -7.3372) (1.1431, -7.3352) (1.18, -7.3282) (1.2249, -7.3213) (1.2695, -7.3132) (1.3067, -7.3078) (1.3324, -7.3011) (1.3463, -7.2942) (1.3565, -7.2875) (1.3658, -7.2796) (1.3741, -7.2706) (1.3818, -7.2601) (1.404, -7.2157) (1.4301, -7.1492) (1.4645, -7.064) (1.491, -6.993) (1.5155, -6.9237) (1.5378, -6.8562) (1.5581, -6.7905) (1.5821, -6.707) (1.598, -6.6449) (1.6076, -6.6042) knots 0.000063 0.000063 0.000063 0.000063 0.072335 0.110531 0.150078 0.190978 0.23323 0.276835 0.321791 0.391759 0.40017 0.407178 0.414186 0.421194 0.428201 0.435209 0.447802 0.473901 0.5 0.526099 0.552198 0.564791 0.571799 0.578806 0.585814 0.592822 0.59983 0.608241 0.678209 0.723165 0.76677 0.809022 0.849922 0.889469 0.927665 0.999937 0.999937 0.999937 0.999937 projected
  arc A25 (1.6076, -6.6042) -> (2.1198, -6.458) centre (0, 0) ccw projected
  spline S25 degree 3 poles (2.1198, -6.458) (2.1494, -6.4876) (2.1956, -6.5319) (2.2601, -6.5902) (2.312, -6.6353) (2.3666, -6.6809) (2.4239, -6.7268) (2.4839, -6.7731) (2.5581, -6.8273) (2.6155, -6.87) (2.6577, -6.896) (2.6698, -6.9009) (2.6816, -6.9042) (2.6936, -6.9059) (2.7058, -6.9062) (2.7213, -6.9048) (2.7467, -6.8969) (2.7811, -6.8819) (2.8233, -6.8652) (2.865, -6.8474) (2.9, -6.8338) (2.9237, -6.8216) (2.9356, -6.8117) (2.9441, -6.8029) (2.9514, -6.7932) (2.9575, -6.7826) (2.9627, -6.7706) (2.9744, -6.7224) (2.9851, -6.6517) (2.9997, -6.561) (3.0097, -6.4859) (3.0182, -6.4129) (3.0249, -6.3421) (3.0301, -6.2736) (3.0349, -6.1867) (3.0366, -6.1227) (3.0368, -6.0809) knots 0.000063 0.000063 0.000063 0.000063 0.072335 0.110531 0.150078 0.190978 0.23323 0.276835 0.321791 0.391759 0.40017 0.407178 0.414186 0.421194 0.428201 0.435209 0.447802 0.473901 0.5 0.526099 0.552198 0.564791 0.571799 0.578806 0.585814 0.592822 0.59983 0.608241 0.678209 0.723165 0.76677 0.809022 0.849922 0.889469 0.927665 0.999937 0.999937 0.999937 0.999937 projected
  arc A26 (3.0368, -6.0809) -> (3.5036, -5.8244) centre (0, 0) ccw projected
  spline S26 degree 3 poles (3.5036, -5.8244) (3.5391, -5.8466) (3.5941, -5.8795) (3.6699, -5.922) (3.7306, -5.9544) (3.7939, -5.9867) (3.86, -6.0188) (3.9288, -6.0506) (4.0132, -6.0869) (4.0786, -6.1158) (4.1256, -6.1317) (4.1385, -6.1338) (4.1506, -6.1344) (4.1628, -6.1334) (4.1748, -6.131) (4.1895, -6.1261) (4.2125, -6.1128) (4.2427, -6.0905) (4.2802, -6.0648) (4.3169, -6.0382) (4.348, -6.0172) (4.3683, -5.9999) (4.3778, -5.9877) (4.3841, -5.9772) (4.3891, -5.9661) (4.3926, -5.9544) (4.395, -5.9416) (4.3957, -5.892) (4.3904, -5.8207) (4.3845, -5.729) (4.3775, -5.6535) (4.3695, -5.5805) (4.3603, -5.51) (4.3501, -5.442) (4.3355, -5.3563) (4.3229, -5.2935) (4.3138, -5.2526) knots 0.000063 0.000063 0.000063 0.000063 0.072335 0.110531 0.150078 0.190978 0.23323 0.276835 0.321791 0.391759 0.40017 0.407178 0.414186 0.421194 0.428201 0.435209 0.447802 0.473901 0.5 0.526099 0.552198 0.564791 0.571799 0.578806 0.585814 0.592822 0.59983 0.608241 0.678209 0.723165 0.76677 0.809022 0.849922 0.889469 0.927665 0.999937 0.999937 0.999937 0.999937 projected
  arc A27 (4.3138, -5.2526) -> (4.7119, -4.8987) centre (0, 0) ccw projected
  spline S27 degree 3 poles (4.7119, -4.8987) (4.7514, -4.9125) (4.8123, -4.9324) (4.8957, -4.9569) (4.962, -4.975) (5.031, -4.9924) (5.1025, -5.0089) (5.1767, -5.0246) (5.2671, -5.0413) (5.3372, -5.0549) (5.3866, -5.06) (5.3996, -5.0591) (5.4116, -5.0569) (5.4233, -5.0533) (5.4344, -5.0483) (5.4476, -5.0403) (5.4672, -5.0221) (5.4916, -4.9937) (5.5224, -4.9603) (5.5523, -4.9262) (5.5779, -4.8988) (5.5939, -4.8775) (5.6004, -4.8634) (5.6042, -4.8518) (5.6066, -4.8399) (5.6075, -4.8277) (5.6069, -4.8146) (5.5966, -4.7661) (5.5756, -4.6978) (5.5494, -4.6098) (5.5258, -4.5377) (5.5017, -4.4683) (5.4771, -4.4016) (5.452, -4.3376) (5.4187, -4.2573) (5.3924, -4.1989) (5.3745, -4.161) knots 0.000063 0.000063 0.000063 0.000063 0.072335 0.110531 0.150078 0.190978 0.23323 0.276835 0.321791 0.391759 0.40017 0.407178 0.414186 0.421194 0.428201 0.435209 0.447802 0.473901 0.5 0.526099 0.552198 0.564791 0.571799 0.578806 0.585814 0.592822 0.59983 0.608241 0.678209 0.723165 0.76677 0.809022 0.849922 0.889469 0.927665 0.999937 0.999937 0.999937 0.999937 projected
  circle A28 centre (0, 0) radius 4.025 projected
  point P0 (0, 0)
extrude "Extrusion2" add sketch "Sketch3" against normal blind 5.08
body "Solid1"
